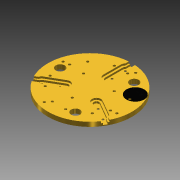
# Autodesk Inventor part: Body
Saved by Autodesk Inventor 2014 (Build 180170000, 170)
## iProperties
Created: 2014-02-04
Part Number: Body
Material: Generic
Document SubType Name: Modeling
Designer: Spooner
Density: 1 g/cm^3
Appearance: Gold - Metal
Author: Spooner
Autodesk Inventor part; units mm, degrees
ref_plane "YZ Plane" through (0, 0, 0) normal (1, 0, 0) x (0, 1, 0)
ref_plane "XZ Plane" through (0, 0, 0) normal (0, 1, 0) x (-1, 0, 0)
ref_plane "XY Plane" through (0, 0, 0) normal (0, 0, 1) x (1, 0, 0)
sketch "Sketch1" plane through (0, 0, 0) normal (0, 1, 0) x (-1, 0, 0)
  circle A0 centre (0, 0) radius 60.325
  dimension "d0" = 120.65
  constraints: 1 centre point, 1 coincident
  measures "d0" diameter of A0
extrude "Extrusion1" add sketch "Sketch1" along normal blind 6.35
sketch "Sketch2" plane through (0, 6.35, 0) normal (0, 1, 0) x (1, 0, 0)
  circle A0 centre (0, 0) radius 60.325 projected
  arc A1 (3.81, 50.8) -> (-3.81, 50.8) centre (0, 50.8) ccw
  arc A2 (-3.81, 25.4) -> (3.81, 25.4) centre (0, 25.4) ccw
  line L0 (-3.81, 50.8) -> (-3.81, 25.4)
  line L1 (3.81, 50.8) -> (3.81, 25.4)
  dimension "d3" = 25.4
  dimension "d4" = 7.62
  dimension "d5" = 50.8
  constraints: 4 end point, 4 point on circle, 4 tangent, 2 centre point, 2 vertical alignment, 1 equal radius
  measures "d3" distance of A1.centre A2.centre
  measures "d4" diameter of A2
  measures "d5" distance of A0.centre A1.centre
extrude "Extrusion2" cut sketch "Sketch2" against normal blind 5.08 contours L1 A2 L0 A1
sketch "Sketch3" plane through (0, 6.35, 0) normal (0, 1, 0) x (1, 0, 0)
  line L0 (-3.81, 25.4) -> (-3.81, 50.8) projected
  arc A0 (3.81, 50.8) -> (-3.81, 50.8) centre (0, 50.8) ccw projected
  line L1 (3.81, 50.8) -> (3.81, 25.4) projected
  arc A1 (-3.81, 25.4) -> (3.81, 25.4) centre (0, 25.4) ccw projected
  line L2 (6.35, 25.4) -> (6.35, 50.8)
  arc A2 (6.35, 50.8) -> (-6.35, 50.8) centre (0, 50.8) ccw
  line L3 (-6.35, 50.8) -> (-6.35, 25.4)
  arc A3 (-6.35, 25.4) -> (6.35, 25.4) centre (0, 25.4) ccw
  dimension "d8" = 2.54
  constraints: 4 end point, 4 point on circle, 2 centre point, 3 other
  measures "d8" distance between parallel lines of L2 L1
extrude "Extrusion3" cut sketch "Sketch3" against normal blind 2.54
sketch "Sketch4" plane through (0, 3.81, 0) normal (0, 1, 0) x (1, 0, 0)
  arc A0 (3.81, 50.8) -> (-3.81, 50.8) centre (0, 50.8) ccw
  line L0 (-2.54, 67.274571) -> (2.54, 67.274571)
  line L1 (2.54, 67.274571) -> (2.54, 48.801843)
  line L2 (2.54, 48.801843) -> (-2.54, 48.801843)
  line L3 (-2.54, 48.801843) -> (-2.54, 67.274571)
  point P0 (0, 0)
  point P1 (0, 48.801843)
  dimension "d11" = 5.08
  constraints: 8 end point, 2 parallel, 1 horizontal, 1 midpoint, 1 perpendicular, 1 vertical alignment
  measures "d11" distance of L1.end L2.end
extrude "Extrusion4" cut sketch "Sketch4" against normal blind 2.54
sketch "Sketch5" plane through (0, 6.35, 0) normal (0, 1, 0) x (1, 0, 0)
  arc A0 (6.35, 50.8) -> (-6.35, 50.8) centre (0, 50.8) ccw
  line L0 (4.445, 43.452518) -> (-4.445, 43.452518)
  line L1 (-4.445, 43.452518) -> (-4.445, 150.339891)
  line L2 (-4.445, 150.339891) -> (4.445, 150.339891)
  line L3 (4.445, 150.339891) -> (4.445, 43.452518)
  point P0 (0, 43.452518)
  dimension "d14" = 8.89
  constraints: 8 end point, 2 parallel, 1 horizontal, 1 midpoint, 1 perpendicular, 1 vertical alignment
  measures "d14" distance of L1.end L2.end
extrude "Extrusion5" cut sketch "Sketch5" against normal blind 2.54
sketch "Sketch6" plane through (0, 1.27, 0) normal (0, 1, 0) x (1, 0, 0)
  arc A0 (-2.54, 53.639806) -> (-3.81, 50.8) centre (0, 50.8) ccw
  arc A1 (-3.81, 25.4) -> (3.81, 25.4) centre (0, 25.4) ccw
  circle A2 centre (0, 50.8) radius 1.524
  circle A3 centre (0, 31.75) radius 1.524
  dimension "d17" = 6.35
  dimension "d18" = 19.05
  dimension "d19" = 3.048
  constraints: 2 centre point, 1 equal radius, 1 vertical alignment
  measures "d17" distance of A1.centre A3.centre
  measures "d18" distance of A2.centre A3.centre
  measures "d19" diameter of A2
extrude "Extrusion6" cut sketch "Sketch6" against normal through all
sketch "Sketch8" plane through (0, 6.35, 0) normal (0, 1, 0) x (1, 0, 0)
  arc A0 (6.35, 50.8) -> (4.445, 55.334807) centre (0, 50.8) ccw
  circle A1 centre (25.4, 38.1) radius 6.35
  dimension "d25" = 12.7
  dimension "d26" = 25.4
  dimension "d27" = 12.7
  constraints: 1 centre point
  measures "d25" diameter of A1
  measures "d26" horizontal distance of A0.centre A1.centre
  measures "d27" vertical distance of A0.centre A1.centre
extrude "Extrusion8" cut sketch "Sketch8" against normal through all
ref_plane "Work Plane1" through (0, 25.4, 25.4) normal (0, 1, 0) x (1, 0, 0)
sketch "Sketch11" plane through (0, 25.4, 25.4) normal (0, 1, 0) x (1, 0, 0)
  circle A0 centre (0, 0) radius 1.7145
  arc A1 (-4.445, 85.561014) -> (4.445, 85.561014) centre (0, 25.4) ccw
  dimension "d41" = 3.429
  dimension "d56" = 25.4
  constraints: 1 centre point, 1 vertical alignment
  measures "d41" diameter of A0
  measures "d56" distance of A0.centre A1.centre
extrude "Extrusion11" cut sketch "Sketch11" against normal through all
pattern_circular "Circular Pattern2" count 3 over 360 about axis through (0, 0, 0) along (0, 1, 0) of "Extrusion2", "Extrusion3", "Extrusion4", "Extrusion5", "Extrusion6", "Extrusion8", "Extrusion11"
sketch "Sketch12" plane through (0, 6.35, 0) normal (0, 1, 0) x (1, 0, 0)
  circle A0 centre (0, -25.4) radius 1.7145 projected
  circle A1 centre (-9.525, -44.45) radius 1.7145
  circle A2 centre (9.525, -44.45) radius 1.7145
  dimension "d47" = 19.05
  dimension "d48" = 9.525
  dimension "d49" = 19.05
  constraints: 2 centre point, 2 equal radius, 1 horizontal alignment
  measures "d47" distance of A2.centre A1.centre
  measures "d48" horizontal distance of A0.centre A1.centre
  measures "d49" vertical distance of A2.centre A0.centre
extrude "Extrusion12" cut sketch "Sketch12" against normal through all contours A1 | A2
pattern_circular "Circular Pattern3" count 6 over 360 about axis through (0, 0, 0) along (0, 1, 0) of "Extrusion12"
sketch "Sketch14" plane through (0, 6.35, 0) normal (0, 1, 0) x (1, 0, 0)
  circle A0 centre (43.257329, 13.976108) radius 1.7145
  circle A1 centre (41.24446, 23.8125) radius 12.7
  arc A2 (54.323466, -26.231024) -> (4.445, 60.161014) centre (0, 0) ccw
  arc A3 (-4.445, 60.161014) -> (-54.323466, -26.231024) centre (0, 0) ccw
  arc A4 (-45.698849, -31.516886) -> (-40.819091, -30.899261) centre (-43.994091, -25.4) ccw
  line L0 (-43.994091, -25.4) -> (71.361423, 41.200537) construction
  dimension "d60" = 25.4
  constraints: 2 end point, 2 point on line, 1 centre point, 1 tangent
  measures "d60" diameter of A1
extrude "Extrusion13" add sketch "Sketch14" along normal blind 0.0508
sketch "Sketch15" plane through (0, 6.35, 0) normal (0, 1, 0) x (1, 0, 0)
  arc A0 (-45.698849, -31.516886) -> (-40.819091, -30.899261) centre (-43.994091, -25.4) ccw
  line L0 (-45.698849, -31.516886) -> (-49.878466, -33.92999)
  arc A1 (-49.878466, -33.92999) -> (49.878466, -33.92999) centre (0, 0) ccw
  circle A2 centre (-14.580568, -50.945716) radius 1.7145
  circle A3 centre (-51.410568, 12.845716) radius 1.7145
  circle A4 centre (14.580568, 50.945716) radius 1.7145
  circle A5 centre (51.410568, -12.845716) radius 1.7145
  line L1 (-43.994091, -25.4) -> (0, 0) construction
  line L2 (14.580568, 50.945716) -> (51.410568, -12.845716) construction
  line L3 (51.410568, -12.845716) -> (-14.580568, -50.945716) construction
  line L4 (-14.580568, -50.945716) -> (-51.410568, 12.845716) construction
  line L5 (-51.410568, 12.845716) -> (14.580568, 50.945716) construction
  line L6 (14.580568, 50.945716) -> (-14.580568, -50.945716) construction
  line L7 (51.410568, -12.845716) -> (-51.410568, 12.845716) construction
  dimension "d63" = 73.66
  dimension "d64" = 3.429
  dimension "d65" = 76.2
  constraints: 14 end point, 4 centre point, 4 coincident, 3 equal radius, 3 parallel, 2 midpoint, 2 perpendicular
  measures "d63" distance of L3.end L4.end
  measures "d64" diameter of A2
  measures "d65" distance of L2.end L3.end
extrude "Extrusion14" cut sketch "Sketch15" against normal through all
equation "\"d48\" = 0.5 * d47"
body "Solid1"
